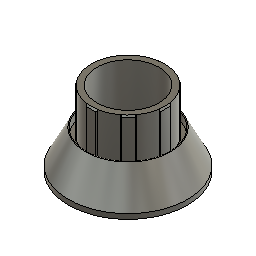
Fuß Tisch Keller (Autodesk Fusion 360 design; units mm, degrees)
Autodesk Fusion 360 part; units mm, degrees
sketch "Skizze1" plane through (0, 0, 0) normal (1, 0, 0) x (0, 0, -1)
  line L0 (0, 0) -> (-25, 0)
  line L1 (-25, 0) -> (-16.8, 16)
  line L2 (-16.8, 16) -> (-16.8, 12)
  line L3 (-16.8, 12) -> (-14.8, 12)
  line L4 (-14.8, 12) -> (-14.8, 30)
  line L5 (-14.8, 30) -> (-12.5, 30)
  line L6 (-12.5, 30) -> (-12.5, 3)
  arc A0 (-12.5, 3) -> (-11.5, 2) centre (-11.5, 3) ccw
  line L7 (-11.5, 2) -> (0, 2)
  line L8 (0, 2) -> (0, 0)
  line L9 (-23.975, 2) -> (-23.975, 0)
  dimension "d1" = 30
  dimension "d2" = 18
  dimension "d3" = 12.5
  dimension "d4" = 2
  dimension "d5" = 14.8
  dimension "d6" = 14
  dimension "d7" = 1
  dimension "d8" = 28
  dimension "d9" = 25
  dimension "d10" = 2
  constraint coincident L0.start L8.end
  constraint horizontal L0
  constraint vertical L2
  constraint perpendicular L2 L3
  constraint perpendicular L3 L4
  constraint perpendicular L2 L5
  constraint perpendicular L5 L6
  constraint tangent L6 A0
  constraint tangent A0 L7
  constraint perpendicular L6 L7
  constraint perpendicular L0 L8
  constraint coincident L1 L9.start
  constraint coincident L0 L9.end
  constraint perpendicular L0 L9
  measures "d1" vertical distance of L0.start L4.end
  measures "d2" distance of L3.end L4.end
  measures "d3" horizontal distance of L0.start L5.end
  measures "d4" distance of L2.end L3.end
  measures "d5" horizontal distance of L0.start L4.end
  measures "d6" vertical distance of L1.end L4.end
  measures "d7" radius of A0
  measures "d8" vertical distance of L5.end L7.end
  measures "d9" distance of L0.start L0.end
  measures "d10" distance of L9.start L9.end
revolve "Drehen1" add sketch "Skizze1" angle 360 about axis through (0, 1.75, 0) along (0, 1, 0) contours L0 L1 L2 L3 L4 L5 L6 A0 L7 L8 L9
fillet "Abrundung1" radius 0.2 1 edges at (-15.6631, 16, 6.0751)
ref_plane "Arbeitsebene1" through (0, 30, 0) normal (0, 1, 0) x (0, 0, 1)
sketch "Skizze2" plane through (0, 30, 0) normal (0, 1, 0) x (1, 0, 0)
  arc A0 (-2, -14.6642) -> (2.2968, -14.6207) centre (0, 0) ccw
  arc A1 (-1.7369, -14.9998) -> (2.0405, -14.9615) centre (0, 0) ccw
  arc A2 (2.0405, -14.9615) -> (2.2968, -14.6207) centre (2, -14.6642) ccw
  arc A3 (-2, -14.6642) -> (-1.7369, -14.9998) centre (-1.7024, -14.7018) ccw
  dimension "d15" = 14.8
  dimension "d16" = 15.1
  dimension "d17" = 4
  dimension "d18" = 2
  constraint coincident A0.centre A1.centre
  constraint tangent A1 A2
  constraint coincident A0.end A2.end
  constraint coincident A0 A2.centre
  constraint tangent A1 A3
  constraint coincident A0 A3.centre
  measures "d15" radius of A0
  measures "d16" radius of A1
  measures "d17" horizontal distance of A0.start A2.centre
  measures "d18" horizontal distance of A0.centre A0.start
extrude "Extrusion1" add sketch "Skizze2" against normal blind 18
sketch "Skizze3" plane through (0, 0, 0) normal (1, 0, 0) x (0, 0, -1)
  line L0 (-14.8, 30) -> (-15.1, 29.1758)
  line L1 (-15.1, 29.1758) -> (-15.1, 30)
  line L2 (-15.1, 30) -> (-14.8, 30)
  dimension "d21" = 14.8
  dimension "d22" = 0.3
  dimension "d23" = 20
  dimension "d24" = 30
  constraint vertical L1
  constraint perpendicular L1 L2
  measures "d21" horizontal distance of origin L0.start
  measures "d22" distance of L0.start L1.end
  measures "d23" angle of L0 L1
  measures "d24" vertical distance of origin L0.start
revolve "Drehen2" cut sketch "Skizze3" angle 360 about axis through (0, 1.75, 0) along (0, 1, 0)
pattern_circular "C-Anordnung1" count 8 over 360 about axis through (0, 1.75, 0) along (0, 1, 0) of "Extrusion1", "Drehen2"
